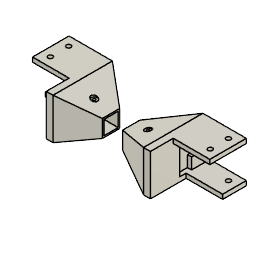
SV08max 1515 holder rev4 (Autodesk Fusion 360 design; units mm, degrees)
Autodesk Fusion 360 part; units mm, degrees
note: some values were not read from the file. Chosen so that the rebuilt part matches the saved one: which sketch regions a step uses; which face or edge a step refers to.
sketch "Skizze1" plane through (0, 0, 0) normal (0, 0, 1) x (1, 0, 0)
  line L0 (0, 0) -> (40, 0)
  line L1 (40, 0) -> (40, 44)
  line L2 (40, 44) -> (0, 44)
  line L3 (0, 44) -> (0, 0)
  circle A0 centre (9.6, 32) radius 2.5
  circle A1 centre (9.6, 12) radius 2.5
  dimension "d1" = 40
  dimension "d2" = 44
  dimension "d5" = 20
  dimension "d6" = 5
  dimension "d7" = 5
  constraint horizontal L0
  constraint vertical L1
  constraint horizontal L2
  constraint vertical L3
  constraint coincident L0.start L3.end
  measures "d1" distance of L0.start L0.end
  measures "d2" distance of L0.start L2.end
  measures "d5" distance of A0.centre A1.centre
  measures "d6" diameter of A0
  measures "d7" diameter of A1
sketch "Skizze2" plane through (0, 0, 0) normal (1, 0, 0) x (0, 1, 0)
  line L0 (44, 0, 40) -> (0, 0, 40)
  line L1 (0, 0, 40) -> (0, -35, 40)
  line L2 (0, -35, 40) -> (44, -35, 40)
  line L3 (44, -35, 40) -> (44, 0, 40)
  point P0 (44, 0)
  dimension "d8" = 44
  dimension "d9" = 35
  measures "d8" distance of P0 origin
sketch "Skizze2 (curves 40 mm off its plane)" plane through (40, 0, 0) normal (1, 0, 0) x (0, 1, 0)
  line L0 (44, 0) -> (0, 0)
  line L1 (0, 0) -> (0, -35)
  line L2 (0, -35) -> (44, -35)
  line L3 (44, -35) -> (44, 0)
extrude "Extrusion1" add sketch "Skizze2 (curves 40 mm off its plane)" along normal blind 5 makes body 1
extrude "Extrusion2" add sketch "Skizze1" along normal blind 5 separate body makes body 2
extrude "Extrusion3" add 1 faces at (40, 14.6667, 1.6667) along direction (1, 0, 0) blind 5 on bodies 2 bodies 1 2
sketch "Skizze3" plane through (0, 0, 0) normal (0, -1, 0) x (1, 0, 0)
  line L0 (40, 0) -> (40, -35)
  line L1 (40, -35) -> (45, -35)
  line L2 (45, -35) -> (45, 5)
  line L3 (45, 5) -> (0, 5)
  line L4 (0, 5) -> (0, 0)
  line L5 (0, 0) -> (40, 0)
  line L6 (45, -35, -44) -> (45, 5, -44)
  line L7 (45, -35, 0) -> (45, -35, -44)
extrude "Extrusion4" cut sketch "Skizze3" against normal blind 2 bodies 1
extrude "Extrusion5" cut 1 faces at (28.3333, 44, 3.3333) along direction (0, -1, 0) blind 2 on bodies 1 bodies 1
sketch "Skizze4" plane through (45, 0, 0) normal (1, 0, 0) x (0, 1, 0)
  line L0 (42, -35) -> (42, 5)
  line L1 (42, 5) -> (2, 5)
  line L2 (2, 5) -> (2, -35)
  line L3 (2, -35) -> (42, -35)
  line L4 (9, -3.4) -> (9, -35)
  line L5 (9, -35) -> (22, -35)
  line L6 (22, -35) -> (22, -3.4)
  line L7 (22, -3.4) -> (9, -3.4)
  constraint vertical L4
  constraint horizontal L5
  constraint vertical L6
  constraint coincident L3 L4.end
  constraint perpendicular L4 L7
extrude "Extrusion6" cut sketch "Skizze4" against normal blind 17 contours L3 L4 L5 L6 L7 bodies 1
extrude "Extrusion7" add sketch "Skizze4" against normal blind 0.5 contours L3 L4 L5 L6 L7 bodies 1
extrude "Extrusion8" add sketch "Skizze4" along normal blind 2 bodies 1
sketch "Skizze5" plane through (47, 0, 0) normal (1, 0, 0) x (0, 1, 0)
  line L0 (2, -35) -> (42, -35)
  line L1 (42, -35) -> (42, 5)
  line L2 (42, 5) -> (2, 5)
  line L3 (2, 5) -> (2, -35)
  line L4 (14.5, -7.5) -> (29.5, -7.5)
  line L5 (29.5, -7.5) -> (29.5, -22.5)
  line L6 (29.5, -22.5) -> (14.5, -22.5)
  line L7 (14.5, -22.5) -> (14.5, -7.5)
  line L8 (31.5, -24.5) -> (12.5, -24.5)
  line L9 (12.5, -24.5) -> (12.5, -5.5)
  line L10 (12.5, -5.5) -> (31.5, -5.5)
  line L11 (31.5, -5.5) -> (31.5, -24.5)
  line L12 (29.5, -22.5, 20) -> (14.5, -22.5, 20)
  line L13 (14.5, -22.5, 20) -> (14.5, -7.5, 20)
  line L14 (29.5, -7.5, 20) -> (29.5, -22.5, 20)
  line L15 (14.5, -7.5, 20) -> (29.5, -7.5, 20)
  line L16 (31.5, -24.5, 20) -> (12.5, -24.5, 20)
  line L17 (12.5, -24.5, 20) -> (12.5, -5.5, 20)
  line L18 (31.5, -5.5, 20) -> (31.5, -24.5, 20)
  line L19 (12.5, -5.5, 20) -> (31.5, -5.5, 20)
  dimension "d33" = 15
  dimension "d34" = 15
  dimension "d37" = -2
  dimension "d39" = 15
  dimension "d40" = 15
  constraint horizontal L4
  constraint vertical L5
  constraint horizontal L6
  constraint vertical L7
  measures "d33" distance of L4.start L4.end
  measures "d34" distance of L4.start L6.end
  measures "d39" distance of L4.start L4.end
  measures "d40" distance of L4.start L6.end
sketch "Skizze5 (curves 20 mm off its plane)" plane through (67, 0, 0) normal (1, 0, 0) x (0, 1, 0)
  line L0 (29.5, -22.5) -> (14.5, -22.5)
  line L1 (14.5, -22.5) -> (14.5, -7.5)
  line L2 (29.5, -7.5) -> (29.5, -22.5)
  line L3 (14.5, -7.5) -> (29.5, -7.5)
  line L4 (31.5, -24.5) -> (12.5, -24.5)
  line L5 (12.5, -24.5) -> (12.5, -5.5)
  line L6 (31.5, -5.5) -> (31.5, -24.5)
  line L7 (12.5, -5.5) -> (31.5, -5.5)
extrude "Extrusion9" add sketch "Skizze5 (curves 20 mm off its plane)" along normal blind 1 separate body makes body 3
loft "Erhebung1" add profiles "Skizze5", "Skizze5 (curves 20 mm off its plane)" section 1 contours L0 L1 L2 L3 | L4 L5 L6 L7 | L8 L9 L10 L11 section 2 bodies 1 3
extrude "Extrusion10" cut sketch "Skizze5 (curves 20 mm off its plane)" against normal blind 72 contours L0 L1 L2 L3 bodies 1
extrude "Extrusion11" cut 1 faces at (68, 30.8333, -17.5) along direction (-1, 0, 0) blind 1 on bodies 1 bodies 1
sketch "Skizze6" plane through (0, 0, 5) normal (0, 0, 1) x (-1, 0, 0)
  line L0 (-47, -42) -> (0, -42)
  line L1 (0, -42) -> (0, -2)
  line L2 (0, -2) -> (-47, -2)
  line L3 (-47, -2) -> (-47, -42)
  circle A0 centre (-9.6, -12) radius 2.5
  circle A1 centre (-9.6, -32) radius 2.5
  circle A2 centre (-57, -22) radius 2.5
  circle A3 centre (-57, -22) radius 6
  circle A4 through (-51, -22, -47) (-60, -16.8038, -47) (-60, -27.1962, -47)
  dimension "d49" = 5
  dimension "d52" = 12
  dimension "d55" = 12
  constraint concentric A2 A3
  measures "d49" diameter of A2
  measures "d52" diameter of A3
extrude "Extrusion12" cut sketch "Skizze6" against normal blind 52 contours A2 bodies 1
extrude "Extrusion13" cut sketch "Skizze6" against normal blind 9 contours A3 bodies 1
sketch "Skizze6 (curves -47 mm off its plane)" plane through (0, 0, -42) normal (0, 0, 1) x (-1, 0, 0)
  circle A0 centre (-57, -22) radius 6
extrude "Extrusion14" cut sketch "Skizze6 (curves -47 mm off its plane)" along normal blind 16 bodies 1
extrude "Extrusion15" cut 1 faces at (52, 14.5, -17.5) along direction (0, -1, 0) blind 0.25 on bodies 1 bodies 1
extrude "Extrusion16" cut 1 faces at (64.5, 21.9167, -7.5) along direction (0, 0, 1) blind 0.25 on bodies 1 bodies 1
extrude "Extrusion17" cut 1 faces at (49, 29.5, -12.3333) along direction (0, 1, 0) blind 0.25 on bodies 1 bodies 1
extrude "Extrusion18" cut 1 faces at (64.5, 22, -22.5) along direction (0, 0, -1) blind 0.25 on bodies 1 bodies 1
sketch "Skizze7" plane through (40, 0, 0) normal (-1, 0, 0) x (0, -1, 0)
  line L0 (-22, -22.75) -> (-29.75, -22.75)
  line L1 (-29.75, -22.75) -> (-29.75, -7.25)
  line L2 (-29.75, -7.25) -> (-22, -7.25)
  line L3 (-22, -7.25) -> (-22, -3.4)
  line L4 (-22, -3.4) -> (-9, -3.4)
  line L5 (-9, -3.4) -> (-9, -35)
  line L6 (-9, -35) -> (-2, -35)
  line L7 (-2, -35) -> (-2, 0)
  line L8 (-2, 0) -> (-42, 0)
  line L9 (-42, 0) -> (-42, -35)
  line L10 (-42, -35) -> (-22, -35)
  line L11 (-22, -35) -> (-22, -22.75)
  line L12 (-14.25, -22.75, -4.5) -> (-29.75, -22.75, -4.5)
  line L13 (-29.75, -22.75, -4.5) -> (-29.75, -7.25, -4.5)
  line L14 (-14.25, -7.25, -4.5) -> (-14.25, -22.75, -4.5)
  line L15 (-29.75, -7.25, -4.5) -> (-14.25, -7.25, -4.5)
  point P0 (-29.75, -7.25)
  point P1 (-14.25, -22.75)
sketch "Skizze7 (curves -4.5 mm off its plane)" plane through (44.5, 0, 0) normal (-1, 0, 0) x (0, -1, 0)
  line L0 (-14.25, -22.75) -> (-29.75, -22.75)
  line L1 (-29.75, -22.75) -> (-29.75, -7.25)
  line L2 (-14.25, -7.25) -> (-14.25, -22.75)
  line L3 (-29.75, -7.25) -> (-14.25, -7.25)
extrude "Extrusion19" add sketch "Skizze7 (curves -4.5 mm off its plane)" against normal blind 5 bodies 1
move_body "Verschieben1" bodies 1 to x (1, 0, 0) y (0, 1, 0) z (0, 0, 1) at (-10, 0, 0)
extrude "Extrusion22" cut 1 faces at (33, 17.6667, -3.4) along direction (0, 0, 1) blind 3.4 on bodies 1 bodies 1
move_body "Verschieben2" bodies 1 to x (1, 0, 0) y (0, 1, 0) z (0, 0, 1) at (-150, 0, 0)
split "Teilen1" by plane through (-115.5, 0, 0) normal (-1, 0, 0) bodies 1 makes body 4 at (-126.3825, 24.9718, 5)
move_body "Verschieben3" bodies 4 to x (1, 0, 0) y (0, 1, 0) z (0, 0, 1) at (-40, 0, 0)
sketch "Skizze8" plane through (-155.5, 0, 0) normal (1, 0, 0) x (0, 1, 0)
  line L0 (9, -35) -> (9, 0)
  line L1 (9, 0) -> (22, 0)
  line L2 (22, 0) -> (22, -7.25)
  line L3 (22, -7.25) -> (29.75, -7.25)
  line L4 (29.75, -7.25) -> (29.75, -22.75)
  line L5 (29.75, -22.75) -> (22, -22.75)
  line L6 (22, -22.75) -> (22, -35)
  line L7 (22, -35) -> (42, -35)
  line L8 (42, -35) -> (42, 5)
  line L9 (42, 5) -> (2, 5)
  line L10 (2, 5) -> (2, -35)
  line L11 (2, -35) -> (9, -35)
  line L12 (42, 5) -> (2, 5)
  line L13 (2, 5) -> (2, -35)
  line L14 (2, -35) -> (42, -35)
  line L15 (42, -35) -> (42, 5)
  constraint horizontal L12
  constraint vertical L13
  constraint horizontal L14
  constraint vertical L15
  constraint coincident L10.end L11.start
  constraint coincident L8.end L9.start
extrude "Extrusion23" add sketch "Skizze8" along normal blind 3 bodies 4
sketch "Skizze9" plane through (-152.5, 0, 0) normal (1, 0, 0) x (0, 1, 0)
  line L0 (42, -35) -> (42, 5)
  line L1 (42, 5) -> (2, 5)
  line L2 (2, 5) -> (2, -35)
  line L3 (2, -35) -> (42, -35)
  line L4 (2, -35) -> (-23, -35)
  line L5 (2, 5) -> (-23, 5)
  line L6 (-23, 5) -> (-23, -35)
  dimension "d78" = 25
  dimension "d79" = 25
  constraint coincident L2.end L3.start
  constraint perpendicular L2 L4
  constraint coincident L1.end L2.start
  constraint perpendicular L2 L5
  measures "d78" distance of L2.end L4.end
  measures "d79" distance of L1.end L5.end
extrude "Extrusion24" add sketch "Skizze9" along normal blind 5 bodies 4
extrude "Extrusion25" add 1 faces at (-152.5, -6.3333, -21.6667) along direction (-1, 0, 0) blind 5 on bodies 4 bodies 4
move_body "Verschieben4" bodies 1 to x (1, 0, 0) y (0, 1, 0) z (0, 0, 1) at (0, -25, 0)
move_body "Verschieben5" bodies 1 to x (1, 0, 0) y (0, 1, 0) z (0, 0, 1) at (-20, 0, 0)
extrude "Extrusion26" cut 1 faces at (-147.5, -1.3333, -21.6667) along direction (-1, 0, 0) blind 5 on bodies 4 bodies 4
sketch "Skizze10" plane through (-113, 0, 0) normal (1, 0, 0) x (0, 1, 0)
  line L0 (4.75, -7.25) -> (4.75, -22.75)
  line L1 (4.75, -22.75) -> (-10.75, -22.75)
  line L2 (-10.75, -7.25) -> (4.75, -7.25)
  line L3 (-12.5, -24.5) -> (6.5, -24.5)
  line L4 (-17.75, -22.75) -> (-2.25, -22.75)
  line L5 (-2.25, -22.75) -> (-2.25, -7.25)
  line L6 (-17.75, -7.25) -> (-17.75, -22.75)
  line L7 (-2.25, -7.25) -> (-17.75, -7.25)
  line L8 (-0.5, -24.5) -> (-19.5, -24.5)
  line L9 (-19.5, -24.5) -> (-19.5, -5.5)
  line L10 (-0.5, -5.5) -> (-0.5, -24.5)
  line L11 (-19.5, -5.5) -> (-0.5, -5.5)
  point P0 (-23, 5)
  point P1 (42, -35)
  constraint horizontal L4
  constraint vertical L5
  constraint horizontal L7
  constraint vertical L6
  constraint horizontal L11
  constraint vertical L10
  constraint horizontal L8
  constraint vertical L9
delete_body "Körper entfernen1" bodies 1
extrude "Extrusion29" add sketch "Skizze10" against normal blind 1 separate body contours L1 L2 L5 L10 | L1 L2 L3 L4 L6 L7 L8 L9 L10 L11 | L1 L2 L4 L5 L6 L7 makes body 5
move_body "Verschieben6" bodies 5 to x (1, 0, 0) y (0, 1, 0) z (0, 0, 1) at (0, 12, 0)
split "Teilen2" by plane through (-160, 0, 0) normal (-1, 0, 0) bodies 4 makes body 6 at (-169.3825, 24.9718, 5)
copy_body "Körper kopieren/einfügen1" bodies 6 makes body 7
move_body "Verschieben7" bodies 7 to x (1, 0, 0) y (0, 1, 0) z (0, 0, 1) at (0, 0, -40)
extrude "Extrusion30" add 1 faces at (-160, 22, -36.6667) along direction (1, 0, 0) blind 7.5 on bodies 7 bodies 4 6 7
sketch "Skizze11" plane through (0, 2, 0) normal (0, -1, 0) x (1, 0, 0)
  line L0 (-160, 5) -> (-160, -35)
  line L1 (-160, -35) -> (-200, -35)
  line L2 (-200, -35) -> (-200, -40)
  line L3 (-200, -40) -> (-152.5, -40)
  line L4 (-152.5, -40) -> (-152.5, -35)
  line L5 (-152.5, -35) -> (-157.5, -35)
  line L6 (-157.5, -35) -> (-157.5, 5)
  line L7 (-157.5, 5) -> (-160, 5)
  line L8 (-160, 5) -> (-157.5, 5)
  line L9 (-157.5, 5) -> (-157.5, -35)
  line L10 (-157.5, -35) -> (-160, -35)
  line L11 (-160, -35) -> (-160, 5)
  line L12 (-200, -35) -> (-157.5, -35)
  line L13 (-157.5, -35) -> (-157.5, -40)
  line L14 (-157.5, -40) -> (-200, -40)
  line L15 (-200, -40) -> (-200, -35)
  constraint horizontal L8
  constraint vertical L9
  constraint horizontal L10
  constraint vertical L11
  constraint coincident L5.end L6.start
  constraint coincident L0.start L7.end
  constraint horizontal L12
  constraint vertical L13
  constraint horizontal L14
  constraint vertical L15
  constraint coincident L3 L13.end
  constraint coincident L1.end L2.start
extrude "Extrusion31" cut sketch "Skizze11" against normal blind 14 contours L1 L2 L3 L10 L12 L13 L14 L15 bodies 4
extrude "Extrusion32" add 1 faces at (-155.8333, 2, -36.6667) along direction (0, -1, 0) blind 25 on bodies 4 bodies 4
loft "Erhebung3" add section 1 face at (-152.5, 9.3333, -10) section 2 face at (-114, 1.1667, -12.4167) on bodies 4 5 bodies 4 5
sketch "Skizze12" plane through (-113, 0, 0) normal (1, 0, 0) x (0, 1, 0)
  line L0 (-7.5, -5.5) -> (-7.5, -24.5)
  line L1 (-7.5, -24.5) -> (11.5, -24.5)
  line L2 (11.5, -24.5) -> (11.5, -5.5)
  line L3 (11.5, -5.5) -> (-7.5, -5.5)
  line L4 (-15.75, -7.25) -> (-0.25, -7.25)
  line L5 (-0.25, -7.25) -> (-0.25, -22.75)
  line L6 (-0.25, -22.75) -> (-15.75, -22.75)
  line L7 (-15.75, -22.75) -> (-15.75, -7.25)
  dimension "d98" = 15.5
  dimension "d99" = 15.5
  constraint horizontal L4
  constraint vertical L5
  constraint horizontal L6
  constraint vertical L7
  measures "d98" distance of L4.start L4.end
  measures "d99" distance of L4.start L6.end
combine "Kombinieren1" operation add target body 4 tool bodies 6
sketch "Skizze13" plane through (0, 0, 5) normal (0, 0, 1) x (-1, 0, 0)
  circle A0 centre (190.4, -12) radius 2.5
  circle A1 centre (190.4, -32) radius 2.5
  line L0 (200, -2) -> (157.5, -2)
  line L1 (157.5, -2) -> (157.5, 23)
  line L2 (157.5, 23) -> (152.5, 23)
  line L3 (152.5, 23) -> (152.5, -42)
  line L4 (152.5, -42) -> (200, -42)
  line L5 (200, -42) -> (200, -2)
  line L6 (113, 7.5, -10.5) -> (113, -11.5, -10.5)
  circle A2 centre (132.5, -2.0008) radius 3.5
  circle A3 centre (132.5, -2.0008) radius 1.5
  circle A4 through (136, -2.0008, -50) (130.75, 1.0303, -50) (130.75, -5.0319, -50)
  dimension "d105" = 7
  dimension "d106" = 3
  dimension "d107" = 7
  constraint concentric A2 A3
  measures "d105" diameter of A2
  measures "d106" diameter of A3
extrude "Extrusion34" cut sketch "Skizze13" against normal blind 70 contours A3 bodies 4
extrude "Extrusion35" cut sketch "Skizze13" against normal blind 6.5 contours A2 bodies 4
sketch "Skizze13 (curves -50 mm off its plane)" plane through (0, 0, -45) normal (0, 0, 1) x (-1, 0, 0)
  circle A0 centre (132.5, -2.0008) radius 3.5
extrude "Extrusion36" cut sketch "Skizze13 (curves -50 mm off its plane)" along normal blind 13.7 bodies 4
extrude "Extrusion37" cut sketch "Skizze13 (curves -50 mm off its plane)" along normal blind 15 bodies 4
sketch "Skizze14" plane through (-113, 0, 0) normal (1, 0, 0) x (0, 1, 0)
  line L0 (-7.5, -5.5) -> (-7.5, -24.5)
  line L1 (-7.5, -24.5) -> (11.5, -24.5)
  line L2 (11.5, -24.5) -> (11.5, -5.5)
  line L3 (11.5, -5.5) -> (-7.5, -5.5)
  line L4 (-5.75, -7.25) -> (9.75, -7.25)
  line L5 (9.75, -7.25) -> (9.75, -22.75)
  line L6 (9.75, -22.75) -> (-5.75, -22.75)
  line L7 (-5.75, -22.75) -> (-5.75, -7.25)
  dimension "d118" = 15.5
  dimension "d119" = 15.5
  constraint horizontal L4
  constraint vertical L5
  constraint horizontal L6
  constraint vertical L7
  measures "d118" distance of L4.start L4.end
  measures "d119" distance of L4.start L6.end
extrude "Extrusion38" cut sketch "Skizze14" against normal blind 35 contours L4 L5 L6 L7 bodies 4
extrude "Extrusion39" add 1 faces at (-157.5, -14.6667, -23.3333) along direction (-1, 0, 0) blind 2.5 on bodies 4 bodies 4
mirror "Spiegeln5" about plane through (-113, 12, 0) normal (1, 0, 0) of bodies 4 makes body 8
move_body "Verschieben11" bodies 8 to x (1, 0, 0) y (0, 1, 0) z (0, 0, 1) at (20, 0, 0)
extrude "Extrusion40" cut 1 faces at (-113, 10.9167, -12.4167) along direction (-1, 0, 0) blind 1 on bodies 4 bodies 4
extrude "Extrusion41" cut 1 faces at (-93, 10.9167, -12.4167) along direction (1, 0, 0) blind 1 on bodies 8 bodies 8
